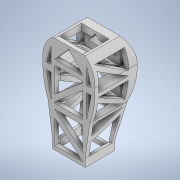
# Autodesk Inventor part: Onderarm(en)
Saved by Autodesk Inventor 2022 (Build 260153000, 153)
## iProperties
Created: 2022-04-25
Part Number: Onderarm(en)
Material: Generic
Document SubType Name: Modeling
Designer: kajve
Density: 1 g/cm^3
Appearance: Default
Author: kajve
Autodesk Inventor part; units mm, degrees
ref_plane "YZ Plane" through (0, 0, 0) normal (1, 0, 0) x (0, 1, 0)
ref_plane "XZ Plane" through (0, 0, 0) normal (0, 1, 0) x (-1, 0, 0)
ref_plane "XY Plane" through (0, 0, 0) normal (0, 0, 1) x (1, 0, 0)
sketch "Sketch1" plane through (0, 0, 0) normal (0, 0, 1) x (1, 0, 0)
  line L0 (0, 0) -> (13.2039, 0)
  line L1 (0, 0) -> (123.8606, 0)
  line L2 (123.8606, 0) -> (123.8606, 288.6967)
  line L3 (123.8606, 288.6967) -> (0, 288.6967)
  line L4 (0, 288.6967) -> (0, 0)
  line L5 (61.9303, 288.6967) -> (61.9303, 0) construction
  circle A0 centre (0, 249.7637) radius 37.033
  arc A1 (-37.033, 249.7637) -> (0, 85.8835) centre (283.6548, 236.107) ccw
  circle A2 centre (123.8606, 249.7637) radius 37.033
  arc A3 (123.8606, 85.8835) -> (160.8936, 249.7637) centre (-159.7941, 236.107) ccw
  line L6 (0, 288.6967) -> (123.8606, 288.6967)
  line L7 (123.8606, 288.6967) -> (123.8606, 338.3523)
  line L8 (123.8606, 338.3523) -> (0, 338.3523)
  line L9 (0, 338.3523) -> (0, 288.6967)
  arc A4 (0, 338.3523) -> (-37.033, 249.7637) centre (65.4631, 258.9518) ccw
  arc A5 (160.8936, 249.7637) -> (123.8606, 338.3523) centre (58.3976, 258.9518) ccw
  line L10 (-17.4646, 124.9573) -> (0, 0)
  line L11 (141.3252, 124.9573) -> (123.8606, 0)
  constraints: 24 end point, 10 point on circle, 5 symmetric about line, 4 centre point, 4 parallel, 3 horizontal, 2 horizontal alignment, 2 midpoint, 2 perpendicular, 2 point on line, 1 vertical, 6 other
extrude "Extrusion1" add sketch "Sketch1" along normal blind 200
sketch "Sketch2" plane through (0, 0, 0) normal (-0.9903737, -0.1384192, 0) x (0, 0, 1)
  line L0 (0, 126.1718) -> (0, 0) projected
  line L1 (0, 0) -> (200, 0) projected
  line L2 (200, 126.1718) -> (200, 0) projected
  line L3 (0, 126.1718) -> (200, 126.1718) projected
sketch "Sketch4" plane through (0, 338.3523, 0) normal (0, 1, 0) x (1, 0, 0)
  line L0 (123.8606, 0) -> (0, 0) projected
  line L1 (0, 0) -> (0, -200) projected
  line L2 (123.8606, -200) -> (0, -200) projected
  line L3 (123.8606, 0) -> (123.8606, -200) projected
  line L4 (0, 0) -> (123.8606, 0)
  line L5 (123.8606, 0) -> (123.8606, -200)
  line L6 (123.8606, -200) -> (0, -200)
  line L7 (0, -200) -> (0, 0)
  constraints: 8 end point, 2 parallel, 1 horizontal, 1 perpendicular
extrude "Extrusion2" add sketch "Sketch4" along normal blind 50
sketch "Sketch5" plane through (0, 338.3523, 200) normal (-1, 0, 0) x (0, 0, 1)
  line L0 (-200, 0) -> (0, 0) projected
  line L1 (0, 0) -> (0, 50) projected
  line L2 (-200, 50) -> (0, 50) projected
  line L3 (-200, 0) -> (-200, 50) projected
  point P0 (-200, -338.3523)
extrude "Extrusion3" add sketch "Sketch5" along normal blind 60
sketch "Sketch6" plane through (-60, 338.3523, 200) normal (-1, 0, 0) x (0, 0, 1)
  line L0 (-200, 0) -> (0, 0) projected
  line L1 (0, 0) -> (0, 50) projected
  line L2 (0, 50) -> (-200, 50) projected
  line L3 (-200, 50) -> (-200, 0) projected
  line L4 (-200, 0) -> (0, 0) projected
  line L5 (-200, -88.5887) -> (0, -88.5887) projected
  line L6 (-200, -213.3951) -> (0, -213.3951) projected
  arc A0 (-132.4552, 0) -> (-160.9091, -88.5887) centre (6.1328, -93.3771) ccw
  line L7 (-200, -338.3523) -> (0, -338.3523) projected
  line L8 (-142.4509, -213.3951) -> (-111.3866, -338.3523)
  line L9 (-111.3866, -338.3523) -> (-200, -338.3523)
  line L10 (-200, -338.3523) -> (-200, -213.3951) projected
  line L11 (-200, -338.3523) -> (-200, -213.3951)
  line L12 (-200, -213.3951) -> (-200, -88.5887)
  line L13 (-200, -88.5887) -> (-200, 0) projected
  line L14 (-200, 0) -> (-200, -88.5887)
  arc A1 (-160.9091, -88.5887) -> (-142.4509, -213.3951) centre (221.9195, -95.7387) ccw
  constraints: 10 end point, 4 point on circle, 4 point on line, 3 collinear, 2 centre point
extrude "Extrusion4" cut sketch "Sketch6" against normal through all
sketch "Sketch7" plane through (0, 0, 200) normal (0, -1, 0) x (1, 0, 0)
  line L0 (0, -111.3866) -> (123.8606, -111.3866) projected
  line L1 (123.8606, -111.3866) -> (123.8606, 0) projected
  line L2 (0, 0) -> (123.8606, 0) projected
  line L3 (0, -111.3866) -> (0, 0) projected
  point P0 (0, -200)
extrude "Extrusion5" add sketch "Sketch7" along normal blind 30
sketch "Sketch9" plane through (0, -30, 200) normal (0, -1, 0) x (1, 0, 0)
  line L0 (123.8606, 0) -> (0, 0) projected
  line L1 (115, 0) -> (8.861, 0)
  line L2 (8.861, 0) -> (8.861, -101.0151)
  line L3 (8.861, -101.0151) -> (115, -101.0151)
  line L4 (115, -101.0151) -> (115, 0)
  point P0 (0, -200)
  dimension "d10" = 106.139
  constraints: 8 end point, 2 parallel, 1 horizontal, 1 perpendicular, 1 point on line
  measures "d10" distance of L3.end L2.end
extrude "Extrusion6" cut sketch "Sketch9" against normal through all
sketch "Sketch10" plane through (123.8606, 0, 88.6134) normal (0, 0, -1) x (-1, 0, 0)
  line L0 (123.8606, 0) -> (0, 0) projected
  line L1 (0, 0) -> (0, -30) projected
  line L2 (123.8606, -30) -> (0, -30) projected
  line L3 (123.8606, 0) -> (123.8606, -30) projected
extrude "Extrusion7" add sketch "Sketch10" along normal blind 50
sketch "Sketch11" plane through (123.8606, 0, 38.6134) normal (0, 0, -1) x (-1, 0, 0)
  line L0 (123.8606, 0) -> (0, 0) projected
  line L1 (0, 0) -> (0, -30) projected
  line L2 (0, -30) -> (123.8606, -30) projected
  line L3 (123.8606, -30) -> (123.8606, 0) projected
  line L4 (114.9996, -30) -> (114.9996, 338.3523) projected
  line L5 (114.9996, -15) -> (8.8606, -15)
  line L6 (0, 0) -> (0, -30) projected
  line L7 (8.8606, -15) -> (8.8606, 75)
  line L8 (8.8606, -30) -> (8.8606, 338.3523) projected
  line L9 (8.8606, 75) -> (114.9996, -15)
  line L10 (114.9996, 15) -> (8.8606, 105)
  line L11 (8.8606, 105) -> (114.9996, 105)
  line L12 (114.9996, 15) -> (114.9996, 105)
  line L13 (114.9996, 130) -> (8.8606, 130)
  line L14 (8.8606, 130) -> (114.9996, 220.0001)
  line L15 (114.9996, 220.0001) -> (114.9996, 130)
  line L16 (114.9996, 245) -> (8.8606, 154.1762)
  line L17 (8.8606, 154.1762) -> (8.8606, 245)
  line L18 (8.8606, 245) -> (114.9996, 245)
  line L19 (160.8936, 249.7637) -> (-37.033, 249.7637) projected
  line L20 (114.9996, 270) -> (8.8606, 270)
  line L21 (8.8606, 270) -> (61.9303, 329.5594)
  line L22 (61.9303, 329.5594) -> (114.9996, 270)
  line L23 (130, 130) -> (147.2707, 220.0001)
  line L24 (141.3252, 124.9573) -> (-17.4646, 124.9573) projected
  line L25 (147.2707, 220.0001) -> (130, 220.0001)
  line L26 (130, 220.0001) -> (130, 130)
  line L27 (147.2707, 245) -> (130, 245)
  line L28 (130, 245) -> (130, 305.2358)
  line L29 (130, 305.2358) -> (147.2707, 245)
  line L30 (8.8606, -30) -> (114.9996, -30) construction
  line L31 (61.9301, -30) -> (61.9303, 338.3523) construction
  line L32 (123.8606, 338.3523) -> (0, 338.3523) construction
  line L33 (-6.1396, 130.0001) -> (-23.4101, 220.0002)
  line L34 (-23.4101, 220.0002) -> (-6.1395, 220.0002)
  line L35 (-6.1395, 220.0002) -> (-6.1396, 130.0001)
  line L36 (-23.4101, 245.0001) -> (-6.1394, 245.0001)
  line L37 (-6.1394, 245.0001) -> (-6.1394, 305.2358)
  line L38 (-6.1394, 305.2358) -> (-23.4101, 245.0001)
  dimension "d15" = 106.139
  dimension "d16" = 90
  dimension "d17" = 139.1599
  dimension "d18" = 139.16
  constraints: 56 end point, 6 symmetric about line, 4 horizontal, 4 point on line, 3 perpendicular, 2 midpoint, 2 vertical, 1 parallel, 15 other
  measures "d15" distance of L5.start L5.end
  measures "d16" distance of L5.end L7.end
  measures "d17" distance of L10.start L10.end
  measures "d18" distance of L13.end L14.end
extrude "Extrusion8" cut sketch "Sketch11" against normal blind 50 contours L3 L2 L4 L0 | L4 L9 L0 | L9 L5 L7 L0 | L4 L2 L8 L5 | L7 L8 L2 L1 L0
extrude "Extrusion9" cut sketch "Sketch11" against normal through all contours L9 L5 L7 L0 | L0 L7 L9 | L10 L11 L4 | L13 L14 L4 | L8 L18 L16 | L20 L21 L22 | L29 L27 L28 L19 | L19 L28 L29 | L37 L36 L38 L19 | L19 L38 L37 | L26 L25 L23 | L33 L34 L35
sketch "Sketch12" plane through (123.8606, -30, 200) normal (1, 0, 0) x (0, 0, -1)
  line L0 (111.3866, 0) -> (111.3866, 30) projected
  line L1 (111.3866, 30) -> (0, 30) projected
  line L2 (0, 30) -> (0, 0) projected
  line L3 (0, 0) -> (111.3866, 0) projected
  line L4 (101.0151, 0) -> (0, 0) projected
  line L5 (111.3866, 30) -> (111.3866, 0) projected
  line L6 (0, 0) -> (111.3866, 0)
  line L7 (111.3866, 0) -> (111.3866, 30)
  line L8 (111.3866, 30) -> (0, 30)
  line L9 (0, 30) -> (0, 0)
  point P0 (200, 30)
  constraints: 8 end point, 2 parallel, 1 horizontal, 1 perpendicular
extrude "Extrusion10" add sketch "Sketch12" along normal blind 50
sketch "Sketch13" plane through (173.8606, -30, 200) normal (1, 0, 0) x (0, 0, -1)
  line L0 (111.3866, 0) -> (111.3866, 30) projected
  line L1 (111.3866, 30) -> (0, 30) projected
  line L2 (0, 30) -> (0, 0) projected
  line L3 (0, 0) -> (111.3866, 0) projected
  line L4 (14.1637, 15.2079) -> (95.5507, 15.2079)
  line L5 (111.3866, 30) -> (111.3866, 15) projected
  line L6 (95.5507, 15.2079) -> (127.5402, 143.8873)
  line L7 (137.4896, 135) -> (115.1156, 45) projected
  line L8 (127.5402, 143.8873) -> (14.1637, 143.8873)
  line L9 (14.1637, 143.8873) -> (14.1637, 15.2079)
  line L10 (142.4509, 154.9573) -> (0, 154.9573) projected
  line L11 (14.1637, 154.9573) -> (127.5402, 154.9573)
  line L12 (127.5402, 154.9573) -> (14.1637, 222.9017)
  line L13 (14.1637, 222.9017) -> (14.1637, 154.9573)
  line L14 (127.5402, 174) -> (14.1637, 241.9444)
  line L15 (14.1637, 241.9444) -> (127.5402, 241.9444)
  line L16 (160.9684, 275.0001) -> (0, 275.0001) projected
  line L17 (127.5402, 241.9444) -> (127.5402, 174)
  line L18 (121.6019, 120) -> (14.1637, 79.8512)
  line L19 (14.1637, 101.5193) -> (127.5402, 143.8873)
  line L20 (14.1637, 257.6686) -> (127.5402, 257.6686)
  line L21 (127.5402, 257.6686) -> (14.1637, 325.613)
  line L22 (14.1637, 325.613) -> (14.1637, 257.6686)
  line L23 (149.7344, 335.2358) -> (0, 335.2358) projected
  line L24 (127.5402, 275.4117) -> (14.1637, 343.3561)
  line L25 (14.1637, 343.3561) -> (127.5402, 343.3561)
  line L26 (127.5402, 343.3561) -> (127.5402, 275.4117)
  point P0 (200, 30)
  point P1 (127.5402, 154.9573)
  point P2 (14.1637, 30)
  point P3 (99.228, 30)
  dimension "d26" = 81.387
  constraints: 36 end point, 11 point on line, 8 perpendicular, 7 parallel, 1 horizontal
  measures "d26" distance of L4.start L4.end
extrude "Extrusion11" cut sketch "Sketch13" against normal blind 50 contours L3 L2 L1 L9 L4 L6 L0 | L6 L4 L9 L1
extrude "Extrusion12" cut sketch "Sketch13" against normal through all contours L1 L9 L18 L6 | L19 L9 L8 | L10 L13 L12 | L14 L15 L17 | L21 L20 L22 L16 | L16 L22 L21 | L26 L24 L23 | L23 L24 L25 L26
sketch "Sketch14" plane through (0, -30, 200) normal (0, -1, 0) x (1, 0, 0)
  line L0 (115, 0) -> (115, -101.0151) projected
  line L1 (8.861, -101.0151) -> (8.861, 0) projected
  line L2 (115, -15) -> (8.861, -15)
  line L3 (8.861, -15) -> (8.861, 0)
  line L4 (8.861, 0) -> (115, 0)
  line L5 (115, 0) -> (115, -15)
  point P0 (0, -200)
  constraints: 8 end point, 2 parallel, 1 horizontal, 1 perpendicular, 1 point on line
extrude "Extrusion13" add sketch "Sketch14" against normal blind 369
sketch "Sketch15" plane through (0, 0, 200) normal (0, 0, 1) x (1, 0, 0)
  line L0 (123.8606, 0) -> (0, 0)
  line L1 (0, 0) -> (0, -30)
  line L2 (0, -30) -> (123.8606, -30)
  line L3 (123.8606, -30) -> (123.8606, 0)
  line L4 (114.9996, -30) -> (114.9996, 338.3523)
  line L5 (114.9996, -15) -> (8.8606, -15)
  line L6 (0, 0) -> (0, -30)
  line L7 (8.8606, -15) -> (8.8606, 75)
  line L8 (8.8606, -30) -> (8.8606, 338.3523)
  line L9 (8.8606, 75) -> (114.9996, -15)
  line L10 (114.9996, 15) -> (8.8606, 105)
  line L11 (8.8606, 105) -> (114.9996, 105)
  line L12 (114.9996, 15) -> (114.9996, 105)
  line L13 (114.9996, 130) -> (8.8606, 130)
  line L14 (8.8606, 130) -> (114.9996, 220.0001)
  line L15 (114.9996, 220.0001) -> (114.9996, 130)
  line L16 (114.9996, 245) -> (8.8606, 154.1762)
  line L17 (8.8606, 154.1762) -> (8.8606, 245)
  line L18 (8.8606, 245) -> (114.9996, 245)
  line L19 (160.8936, 249.7637) -> (-37.033, 249.7637)
  line L20 (114.9996, 270) -> (8.8606, 270)
  line L21 (8.8606, 270) -> (61.9303, 329.5594)
  line L22 (61.9303, 329.5594) -> (114.9996, 270)
  line L23 (130, 130) -> (147.2707, 220.0001)
  line L24 (141.3252, 124.9573) -> (-17.4646, 124.9573)
  line L25 (147.2707, 220.0001) -> (130, 220.0001)
  line L26 (130, 220.0001) -> (130, 130)
  line L27 (147.2707, 245) -> (130, 245)
  line L28 (130, 245) -> (130, 305.2358)
  line L29 (130, 305.2358) -> (147.2707, 245)
  line L30 (8.8606, -30) -> (114.9996, -30) construction
  line L31 (61.9301, -30) -> (61.9303, 338.3523) construction
  line L32 (123.8606, 338.3523) -> (0, 338.3523) construction
  line L33 (-6.1395, 220.0002) -> (-6.1396, 130.0001)
  line L34 (-23.4101, 220.0002) -> (-6.1395, 220.0002)
  line L35 (-6.1396, 130.0001) -> (-23.4101, 220.0002)
  line L36 (-6.1394, 305.2358) -> (-23.4101, 245.0001)
  line L37 (-6.1394, 245.0001) -> (-6.1394, 305.2358)
  line L38 (-23.4101, 245.0001) -> (-6.1394, 245.0001)
  point P0 (114.9996, 249.7637)
  point P1 (8.8606, 249.7637)
  point P2 (8.8606, 124.9573)
  point P3 (114.9996, 124.9573)
  dimension "d33" = 106.139
  dimension "d34" = 90
  dimension "d35" = 139.1599
  dimension "d36" = 139.16
  constraints: 74 end point, 6 symmetric about line, 4 horizontal, 4 point on line, 3 perpendicular, 2 midpoint, 2 vertical, 1 parallel, 19 other
  measures "d33" distance of L5.start L5.end
  measures "d34" distance of L5.end L7.end
  measures "d35" distance of L10.start L10.end
  measures "d36" distance of L13.end L14.end
extrude "Extrusion14" cut sketch "Sketch15" against normal blind 20 contours L9 L5 L7 L0 | L0 L7 L9 | L10 L11 L4 | L24 L8 L13 L4 | L13 L14 L4 | L8 L18 L16 | L18 L8 L19 L4 | L20 L21 L22
body "Solid1"
